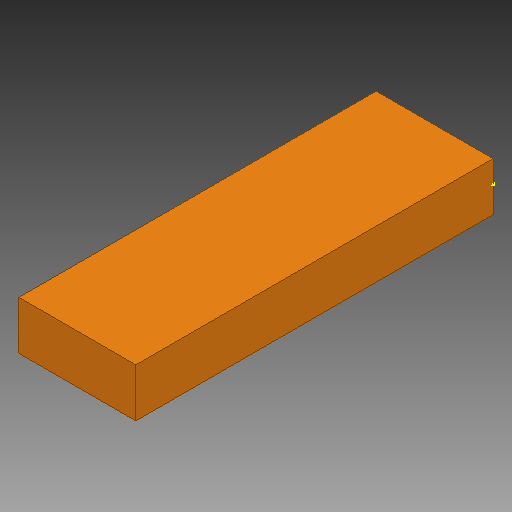
# Autodesk Inventor part: 1x3 short orange smooth
Saved by Autodesk Inventor 2017 (Build 210142000, 142)
## iProperties
Created: 2018-05-10
Part Number: 1x3 short orange smooth
Material: ABS Plastic
Document SubType Name: Modeling
Designer: 20000650
Density: 1.06 g/cm^3
Appearance: Orange
Mass: 0.468139 g
Surface Area: 7.1277 cm^2
Volume: 0.44164 cm^3
Author: 20000650
Autodesk Inventor part; units mm, degrees
ref_plane "YZ Plane" through (0, 0, 0) normal (1, 0, 0) x (0, 1, 0)
ref_plane "XZ Plane" through (0, 0, 0) normal (0, 1, 0) x (-1, 0, 0)
ref_plane "XY Plane" through (0, 0, 0) normal (0, 0, 1) x (1, 0, 0)
sketch "Sketch1" plane through (0, 0, 0) normal (0, 1, 0) x (-1, 0, 0)
  line L0 (0, 0) -> (0, -23.8252)
  line L1 (0, -23.8252) -> (7.7978, -23.8252)
  line L2 (7.7978, -23.8252) -> (7.7978, 0)
  line L3 (7.7978, 0) -> (0, 0)
  dimension "d0" = 23.8252
  dimension "d1" = 7.7978
  constraints: 8 end point, 3 perpendicular, 1 vertical
  measures "d0" distance of L0.start L0.end
  measures "d1" distance of L0.end L1.end
extrude "Extrusion1" add sketch "Sketch1" along normal blind 3.236
shell "Shell1" thickness 1.4732 removed faces 1 at (-2.5993, 3.236, -7.9417)
sketch "Sketch3" plane through (-6.3246, 1.4732, -22.352) normal (0, 1, 0) x (1, 0, 0)
  point P0 (6.3246, -22.352)
sketch "Sketch4" plane through (-6.3246, 1.4732, -22.352) normal (0, 1, 0) x (1, 0, 0)
  line L0 (6.3246, -22.352) -> (2.4257, -22.352) construction
  line L1 (2.4257, -22.352) -> (2.4257, -18.4531) construction
  line L2 (2.4257, -18.4531) -> (6.3246, -18.4531) construction
  line L3 (6.3246, -18.4531) -> (6.3246, -22.352) construction
  circle A0 centre (2.4257, -18.4531) radius 2.4498 construction
  circle A1 centre (2.4257, -10.6553) radius 2.4498 construction
  line L4 (2.4257, -18.4531) -> (2.4257, -10.6553) construction
  circle A2 centre (2.4257, -14.5542) radius 1.4491
  circle A3 centre (2.4257, -14.5542) radius 0.6198
  dimension "d5" = 3.8989
  dimension "d6" = 3.8989
  dimension "d7" = 4.8997
  dimension "d10" = 7.7978
  dimension "d15" = 1.2395
  constraints: 10 end point, 4 centre point, 2 coincident, 2 parallel, 2 vertical, 1 horizontal, 1 midpoint, 1 perpendicular, 2 other
  measures "d5" distance of L1.end L2.end
  measures "d6" distance of L0.end L1.end
  measures "d7" diameter of A0
  measures "d10" distance of L4.start L4.end
  measures "d15" diameter of A3
extrude "Extrusion2" add sketch "Sketch4" along normal up to surface (1.7628 mm away)
pattern_linear "Rectangular Pattern1" count 2 spacing 7.7978 along (0, 0, -1) of "Extrusion2"
body "Solid1"
